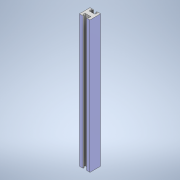
# Autodesk Inventor part: Perfil
Saved by Autodesk Inventor 2021 (Build 250183000, 183)
## iProperties
Created: 2022-01-21
Part Number: Perfil
Material: Generic
Document SubType Name: Modeling
Designer: deuts
Density: 1 g/cm^3
Appearance: Default
Author: deuts
Autodesk Inventor part; units mm, degrees
ref_plane "YZ Plane" through (0, 0, 0) normal (1, 0, 0) x (0, 1, 0)
ref_plane "XZ Plane" through (0, 0, 0) normal (0, 1, 0) x (-1, 0, 0)
ref_plane "XY Plane" through (0, 0, 0) normal (0, 0, 1) x (1, 0, 0)
sketch "Sketch1" plane through (0, 0, 0) normal (0, 1, 0) x (-1, 0, 0)
  line L0 (10, 10) -> (10, -10)
  line L1 (-10, -10) -> (-10, 10)
  line L2 (3.125, -10) -> (3.125, -8.2)
  line L3 (3.125, -8.2) -> (5.5, -8.2)
  line L4 (5.5, -8.2) -> (5.5, -3.9)
  line L5 (5.5, -3.9) -> (-5.5, -3.9)
  line L6 (-5.5, -3.9) -> (-5.5, -8.2)
  line L7 (-5.5, -8.2) -> (-3.125, -8.2)
  line L8 (-3.125, -8.2) -> (-3.125, -10)
  line L9 (10, -10) -> (3.125, -10)
  line L10 (-3.125, -10) -> (-10, -10)
  line L11 (3.125, 10) -> (3.125, 8.2)
  line L12 (3.125, 8.2) -> (5.5, 8.2)
  line L13 (5.5, 8.2) -> (5.5, 3.9)
  line L14 (5.5, 3.9) -> (-5.5, 3.9)
  line L15 (-5.5, 3.9) -> (-5.5, 8.2)
  line L16 (-5.5, 8.2) -> (-3.125, 8.2)
  line L17 (-3.125, 8.2) -> (-3.125, 10)
  line L18 (-10, 10) -> (-3.125, 10)
  line L19 (3.125, 10) -> (10, 10)
  point P0 (0, 0)
  dimension "d0" = 20
  dimension "d1" = 20
  dimension "d4" = 2.375
  dimension "d5" = 4.3
  dimension "d6" = 11
  dimension "d7" = 2.375
  dimension "d8" = 1.8
  dimension "d9" = 6.875
  dimension "d10" = 1.8
  dimension "d11" = 4.3
  constraints: 40 end point, 13 perpendicular, 5 parallel, 2 horizontal, 2 point on line, 2 vertical
  measures "d0" distance of L0.end L1.start
  measures "d1" distance of L0.start L0.end
  measures "d4" distance of L2.end L3.end
  measures "d5" distance of L3.end L4.end
  measures "d6" distance of L4.end L5.end
  measures "d7" distance of L6.end L7.end
  measures "d8" distance of L2.start L2.end
  measures "d9" distance of L0.end L2.start
  measures "d10" distance of L11.start L11.end
  measures "d11" distance of L12.end L13.end
extrude "Extrusion1" add sketch "Sketch1" along normal blind 250
body "Solid1"
